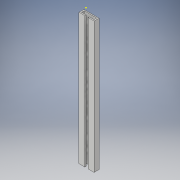
# Autodesk Inventor part: crossbowtrack
Saved by Autodesk Inventor 2018 (Build 220112000, 112)
## iProperties
Created: 2019-02-25
Part Number: crossbowtrack
Material: Generic
Document SubType Name: Modeling
Designer: F8PLTW
Density: 1 g/cm^3
Appearance: Default
Author: F8PLTW
Autodesk Inventor part; units mm, degrees
ref_plane "YZ Plane" through (0, 0, 0) normal (1, 0, 0) x (0, 1, 0)
ref_plane "XZ Plane" through (0, 0, 0) normal (0, 1, 0) x (-1, 0, 0)
ref_plane "XY Plane" through (0, 0, 0) normal (0, 0, 1) x (1, 0, 0)
sketch "Sketch1" plane through (0, 0, 0) normal (0, 0, 1) x (1, 0, 0)
  line L0 (-15.9487, -92.7565) -> (47.5513, -92.7565)
  line L1 (47.5513, -92.7565) -> (47.5513, -346.7565)
  line L2 (47.5513, -346.7565) -> (-15.9487, -346.7565)
  line L3 (-15.9487, -346.7565) -> (-15.9487, -92.7565)
  point P0 (0, 0)
  dimension "d0" = 63.5
  dimension "d2" = 254
  constraints: 8 end point, 2 parallel, 1 horizontal, 1 perpendicular
  measures "d0" distance of L1.end L2.end
  measures "d2" distance of L0.end L1.end
extrude "Extrusion1" add sketch "Sketch1" along normal blind 19.05
sketch "Sketch2" plane through (-15.9487, -92.7565, 0) normal (0, 1, 0) x (1, 0, 0)
  point P0 (15.9487, 0)
sketch "Sketch3" plane through (-15.9487, -92.7565, 0) normal (0, 1, 0) x (1, 0, 0)
  line L0 (63.5, -19.05) -> (0, -19.05) projected
  line L1 (34.925, -19.05) -> (28.575, -19.05)
  line L2 (28.575, -19.05) -> (28.575, -12.0642)
  line L3 (34.925, -12.0642) -> (34.925, -19.05)
  line L4 (31.75, -19.05) -> (31.75, 0) construction
  line L5 (63.5, 0) -> (63.5, -19.05) projected
  line L6 (28.575, -12.0642) -> (19.685, -12.0642)
  line L7 (19.685, -12.0642) -> (19.685, -6.9842)
  line L8 (19.685, -6.9842) -> (28.575, -6.9842)
  line L9 (34.925, -12.0642) -> (43.815, -12.0642)
  line L10 (43.815, -12.0642) -> (43.815, -6.9842)
  line L11 (43.815, -6.9842) -> (34.925, -6.9842)
  line L12 (34.925, -6.9842) -> (28.575, -6.9842)
  point P0 (15.9487, 0)
  dimension "d6" = 31.75
  dimension "d7" = 8.89
  dimension "d8" = 5.08
  dimension "d9" = 8.89
  constraints: 22 end point, 4 horizontal, 4 perpendicular, 3 parallel, 2 point on line, 1 midpoint, 1 other
  measures "d6" distance between parallel lines of L5 L4
  measures "d7" distance of L7.end L8.end
  measures "d8" distance of L6.end L7.end
  measures "d9" distance of L11.end L10.end
extrude "Extrusion2" cut sketch "Sketch3" against normal blind 254
sketch "Sketch4" plane through (-15.9487, -92.7565, 0) normal (0, 1, 0) x (1, 0, 0)
  line L0 (63.5, 0) -> (63.5, -19.05) projected
  line L1 (63.5, 0) -> (46.4201, 0)
  line L2 (46.4201, 0) -> (46.4201, -19.05)
  line L3 (46.4201, -19.05) -> (63.5, -19.05)
  line L4 (63.5, -19.05) -> (63.5, 0)
  line L5 (63.5, 0) -> (0, 0) projected
  line L6 (31.75, 0) -> (31.75, -19.05) construction
  line L7 (0, 0) -> (0, -19.05)
  line L8 (0, 0) -> (17.0799, 0)
  line L9 (17.0799, 0) -> (17.0799, -19.05)
  line L10 (0, -19.05) -> (17.0799, -19.05)
  point P0 (15.9487, 0)
  constraints: 18 end point, 3 symmetric about line, 2 horizontal, 2 parallel, 1 midpoint, 1 perpendicular, 1 vertical
extrude "Extrusion3" cut sketch "Sketch4" against normal blind 254
sketch "Sketch5" plane through (3.7363, -92.7565, 6.9842) normal (0, 1, 0) x (1, 0, 0)
  line L0 (-2.6051, 6.9842) -> (-2.6051, -12.0658) projected
  line L1 (26.7351, 6.9842) -> (26.7351, -12.0658) projected
  line L2 (-2.6051, 6.9842) -> (26.7351, 6.9842)
  line L3 (26.7351, 6.9842) -> (26.7351, 2.1306)
  line L4 (26.7351, 2.1306) -> (-2.6051, 2.1306)
  line L5 (-2.6051, 2.1306) -> (-2.6051, 6.9842)
  point P0 (-3.7363, 6.9842)
  constraints: 8 end point, 2 parallel, 1 horizontal, 1 perpendicular, 1 point on line
extrude "Extrusion4" cut sketch "Sketch5" against normal blind 254
sketch "Sketch6" plane through (3.7363, -92.7565, 6.9842) normal (0, 1, 0) x (1, 0, 0)
  line L0 (-2.6051, -12.0658) -> (-2.6051, 2.1306) projected
  line L1 (26.7351, 2.1306) -> (26.7351, -12.0658) projected
  line L2 (-2.6051, -12.0658) -> (26.7351, -12.0658)
  line L3 (26.7351, -12.0658) -> (26.7351, -7.5248)
  line L4 (26.7351, -7.5248) -> (-2.6051, -7.5248)
  line L5 (-2.6051, -7.5248) -> (-2.6051, -12.0658)
  point P0 (-3.7363, 6.9842)
  constraints: 8 end point, 2 parallel, 1 horizontal, 1 perpendicular, 1 point on line
extrude "Extrusion5" cut sketch "Sketch6" against normal blind 254
body "Solid1"
